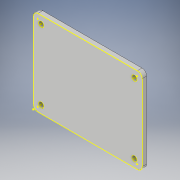
# Autodesk Inventor part: BasePixhawk
Saved by Autodesk Inventor 2019 (Build 230136000, 136)
## iProperties
Created: 2019-02-06
Part Number: BasePixhawk
Material: Generic
Document SubType Name: Modeling
Designer: Kenny
Density: 1 g/cm^3
Appearance: Default
Author: Kenny
Autodesk Inventor part; units mm, degrees
ref_plane "YZ Plane" through (0, 0, 0) normal (1, 0, 0) x (0, 1, 0)
ref_plane "XZ Plane" through (0, 0, 0) normal (0, 1, 0) x (-1, 0, 0)
ref_plane "XY Plane" through (0, 0, 0) normal (0, 0, 1) x (1, 0, 0)
sketch "Sketch1" plane through (0, 0, 0) normal (0, 0, 1) x (1, 0, 0)
  line L0 (0, 0) -> (70, 0)
  line L1 (70, 0) -> (70, 55)
  line L2 (70, 55) -> (0, 55)
  line L3 (0, 55) -> (0, 0)
  point P0 (5, 50)
  point P1 (65, 50)
  point P2 (65, 5)
  point P3 (5, 5)
  dimension "d0" = 70
  dimension "d1" = 55
  dimension "d13" = 5
  dimension "d14" = 5
  dimension "d18" = 60
  dimension "d19" = 45
  constraints: 8 end point, 2 horizontal alignment, 2 parallel, 2 vertical alignment, 1 horizontal, 1 perpendicular
  measures "d0" distance of L2.end L1.end
  measures "d1" distance of L1.end L0.end
  measures "d13" distance from line of L2 point (5, 50)
  measures "d14" distance from line of L3 point (5, 50)
  measures "d18" distance of point (5, 5) point (65, 5)
  measures "d19" distance of point (65, 50) point (65, 5)
extrude "Extrusion1" add sketch "Sketch1" along normal blind 3
sketch "Sketch3" plane through (0, 0, 0) normal (0, 0, 1) x (1, 0, 0)
  line L0 (0, 0) -> (70, 0)
  line L1 (70, 0) -> (70, 55)
  line L2 (70, 55) -> (0, 55)
  line L3 (0, 55) -> (0, 0)
  point P0 (5, 50)
  point P1 (65, 50)
  point P2 (65, 5)
  point P3 (5, 5)
  dimension "d20" = 70
  dimension "d21" = 55
  dimension "d22" = 5
  dimension "d23" = 5
  dimension "d24" = 60
  dimension "d25" = 45
  constraints: 8 end point, 2 horizontal alignment, 2 parallel, 2 vertical alignment, 1 horizontal, 1 perpendicular
  measures "d20" distance of L2.end L1.end
  measures "d21" distance of L1.end L0.end
  measures "d22" distance from line of L2 point (5, 50)
  measures "d23" distance from line of L3 point (5, 50)
  measures "d24" distance of point (5, 5) point (65, 5)
  measures "d25" distance of point (65, 50) point (65, 5)
hole "Hole1" at (5, 50, 0) at (65, 50, 0) at (65, 5, 0) at (5, 5, 0) direction (0, 0, 1) diameter 3.3 end through all
fillet "Fillet1" radius 3 4 edges at (70, 55, 1.5) (70, 0, 1.5) (0, 0, 1.5) (0, 55, 1.5)
sketch "Sketch4" plane through (0, 0, 3) normal (0, 0, 1) x (1, 0, 0)
  arc A0 (3, 55) -> (0, 52) centre (3, 52) ccw projected
  line L0 (0, 52) -> (0, 3) projected
  arc A1 (0, 3) -> (3, 0) centre (3, 3) ccw projected
  line L1 (3, 0) -> (67, 0) projected
  arc A2 (67, 0) -> (70, 3) centre (67, 3) ccw projected
  line L2 (70, 3) -> (70, 52) projected
  arc A3 (70, 52) -> (67, 55) centre (67, 52) ccw projected
  line L3 (67, 55) -> (3, 55) projected
  circle A4 centre (65, 5) radius 1.65 projected
  circle A5 centre (5, 50) radius 1.65 projected
  circle A6 centre (65, 50) radius 1.65 projected
  circle A7 centre (5, 5) radius 1.65 projected
  point P0 (0, 0)
body "Solid1"
